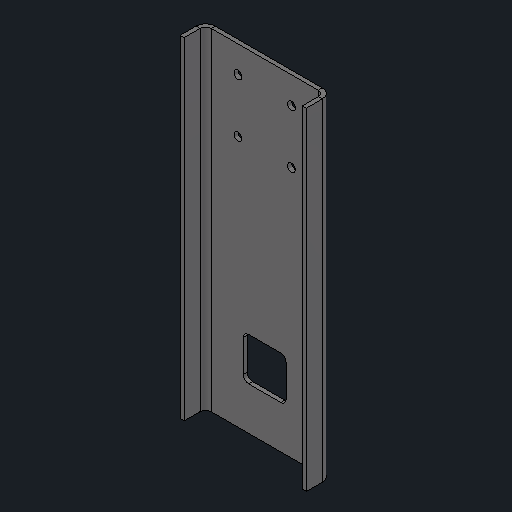
# Autodesk Inventor part: Model-5_Sheet-LH
Saved by Autodesk Inventor 2025.1 (Build 291241000, 241)
## iProperties
RuleStatus: InUse
Created: 2026-02-13
Part Number: Model-5_Sheet-LH
User Status: Released
Material: SS304
Document SubType Name: Sheet Metal
Designer: Desktop -24
Density: 7.99949 g/cm^3
Sheet Metal Rule: 3/8" (3.150 Die)
Appearance: Semi-Polished(1)
AfterDocNew0: Mat. Selection
encoded128: ÌSheet Metal (in)XÎ
Family: SS304
Author: Desktop -24
Revision Number: 0
Autodesk Inventor part; units mm, degrees
ref_plane "YZ Plane" through (0, 0, 0) normal (1, 0, 0) x (0, 1, 0)
ref_plane "XZ Plane" through (0, 0, 0) normal (0, 1, 0) x (-1, 0, 0)
ref_plane "XY Plane" through (0, 0, 0) normal (0, 0, 1) x (1, 0, 0)
sketch "Sketch1" plane through (0, 0, 0) normal (0, 0, 1) x (1, 0, 0)
  line L0 (-127, 0) -> (127, 0)
  line L1 (-127, -787.4) -> (-127, 0)
  line L2 (127, 0) -> (127, -787.4)
  line L3 (-63.5, -190.5) -> (63.5, -190.5) construction
  line L4 (63.5, -190.5) -> (63.5, -63.5) construction
  line L5 (63.5, -63.5) -> (-63.5, -63.5) construction
  line L6 (-63.5, -63.5) -> (-63.5, -190.5) construction
  line L7 (-63.5, -190.5) -> (63.5, -63.5) construction
  line L8 (63.5, -190.5) -> (-63.5, -63.5) construction
  circle A0 centre (-63.5, -63.5) radius 9.525
  circle A1 centre (63.5, -63.5) radius 9.525
  circle A2 centre (63.5, -190.5) radius 9.525
  circle A3 centre (-63.5, -190.5) radius 9.525
  line L9 (-127, -787.4) -> (127, -787.4)
  point P0 (0, 0)
  point P1 (0, 0)
  point P2 (0, -127)
  point P3 (0, -63.5)
  dimension "d1" = 254
  dimension "d7" = 19.05
  dimension "d8" = 127
  dimension "d9" = 127
  dimension "d10" = 63.5
  measures "d1" distance of L0.end L0.start
  measures "d7" diameter of A1
  measures "d8" distance of L4.end L5.end
  measures "d9" distance of L5.end L3.start
  measures "d10" distance between parallel lines of L0 L5
extrude "Plate1" add sketch "Sketch1" along normal blind 9.525
sketch "Sketch3" plane through (-140.208, -787.4, 22.733) normal (-1, 0, 0) x (0, -1, 0)
  line L0 (-787.4, 0) -> (0, 0)
  line L1 (0, 0) -> (0, 37.592)
  line L2 (0, 37.592) -> (-787.4, 37.592)
  line L3 (-787.4, 37.592) -> (-787.4, 0)
  constraints: 6 end point, 1 horizontal, 1 perpendicular, 1 vertical
edge flange "Flange2" height 50.8 angle 90 thickness 9.525 bend radius 13.208 thickness toward (-1, 0, 0) relief tear relief width 9.525 relief depth 4.7625 corner gap 9.525 corner form 0 edges at (-127, -393.7, 9.525) (127, -393.7, 9.525) wall of the first edge with corners at (-140.208, 0, 22.733) (-140.208, -787.4, 22.733) (-140.208, -787.4, 60.325) (-140.208, 0, 60.325)
bend "Bend2"
corner "Corner2"
sketch "Sketch4" plane through (0, 0, 0) normal (0, 0, -1) x (-1, 0, 0)
  line L0 (-38.1, -584.2) -> (38.1, -584.2)
  line L1 (50.8, -596.9) -> (50.8, -673.1)
  line L2 (38.1, -685.8) -> (-38.1, -685.8)
  line L3 (-50.8, -673.1) -> (-50.8, -596.9)
  line L4 (-50.8, -584.2) -> (50.8, -685.8) construction
  line L5 (50.8, -584.2) -> (-50.8, -685.8) construction
  line L6 (127, -787.4) -> (-127, -787.4) projected
  line L7 (-127, 0) -> (127, 0) projected
  arc A0 (-38.1, -584.2) -> (-50.8, -596.9) centre (-38.1, -596.9) ccw
  arc A1 (50.8, -596.9) -> (38.1, -584.2) centre (38.1, -596.9) ccw
  arc A2 (38.1, -685.8) -> (50.8, -673.1) centre (38.1, -673.1) ccw
  arc A3 (-50.8, -673.1) -> (-38.1, -685.8) centre (-38.1, -673.1) ccw
  point P0 (0, 0)
  point P1 (0, -635)
  point P2 (0, 0)
  dimension "d40" = 101.6
  dimension "d41" = 101.6
  dimension "d42" = 101.6
  dimension "d43" = 12.7
  constraints: 12 end point, 8 point on circle, 8 point on line, 8 tangent, 4 centre point, 3 equal radius, 3 midpoint, 2 parallel, 1 horizontal, 1 perpendicular, 1 vertical alignment
  measures "d40" distance of L4.start L5.start
  measures "d41" distance of L5.start L4.end
  measures "d42" distance between parallel lines of L6 L2
  measures "d43" radius of A0
extrude "Cut1" cut sketch "Sketch4" against normal blind 9.525
equation "\"d44\" = Thickness"
equation "\"d15\" = Thickness"
equation "\"d30\" = BendReliefWidth"
equation "\"d31\" = BendReliefDepth"
equation "\"d32\" = MinimumRemnant"
equation "\"d33\" = TransitionRadius"
equation "\"d36\" = BendRadius"
equation "\"d37\" = CornerReliefSize"
equation "\"d38\" = GapSize"
equation "\"d39\" = JacobiRadiusSize"
equation "\"BendReliefWidth\" = Thickness"
equation "\"BendReliefDepth\" = 0.5 * Thickness"
equation "\"CornerReliefSize\" = 4 * Thickness"
equation "\"MinimumRemnant\" = 2 * Thickness"
equation "\"TransitionRadius\" = BendRadius"
equation "\"JacobiRadiusSize\" = Thickness"
equation "\"GapSize\" = Thickness"
equation "\"Thickness\" = 9.525"
equation "\"BendRadius\" = 13.208"
body "Solid1"
